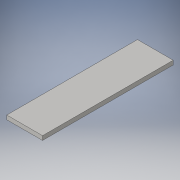
# Autodesk Inventor part: Caster Block
Saved by Autodesk Inventor 2016 (Build 200138000, 138)
## iProperties
Created: 2017-12-23
Part Number: Caster Block
Material: Generic
Document SubType Name: Modeling
Designer: mathaetaes
Density: 1 g/cm^3
Appearance: Default
Author: mathaetaes
Autodesk Inventor part; units mm, degrees
ref_plane "YZ Plane" through (0, 0, 0) normal (1, 0, 0) x (0, 1, 0)
ref_plane "XZ Plane" through (0, 0, 0) normal (0, 1, 0) x (-1, 0, 0)
ref_plane "XY Plane" through (0, 0, 0) normal (0, 0, 1) x (1, 0, 0)
sketch "Sketch1" plane through (0, 0, 0) normal (0, 1, 0) x (-1, 0, 0)
  line L0 (0, 0) -> (-165.1, 0)
  line L1 (-165.1, 0) -> (-165.1, -603.25)
  line L2 (-165.1, -603.25) -> (0, -603.25)
  line L3 (0, -603.25) -> (0, 0)
  dimension "d1" = 603.25
  dimension "d4" = 165.1
  constraints: 8 end point, 2 parallel, 1 horizontal, 1 perpendicular
  measures "d1" distance of L1.end L0.end
  measures "d4" distance of L1.end L2.end
extrude "Board" add sketch "Sketch1" along normal blind 19.05
body "Solid1"
